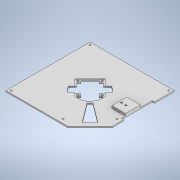
# Autodesk Inventor part: Drop_Plate
Saved by Autodesk Inventor 2022 (Build 260153000, 153)
## iProperties
Created: 2023-02-27
Part Number: Drop_Plate
Material: Generic
Document SubType Name: Modeling
Designer: zarek
Density: 1 g/cm^3
Appearance: Default
Author: zarek
Autodesk Inventor part; units mm, degrees
ref_plane "YZ Plane" through (0, 0, 0) normal (1, 0, 0) x (0, 1, 0)
ref_plane "XZ Plane" through (0, 0, 0) normal (0, 1, 0) x (-1, 0, 0)
sketch "Sketch1" plane through (0, 0, 0) normal (0, 1, 0) x (-1, 0, 0)
  line L0 (101.6, -101.6) -> (-101.6, -101.6)
  line L1 (-101.6, -101.6) -> (-101.6, 101.6)
  line L2 (-101.6, 101.6) -> (101.6, 101.6)
  line L3 (101.6, 101.6) -> (101.6, -101.6)
  line L4 (96.6, -96.6) -> (-96.6, -96.6)
  line L5 (-96.6, -96.6) -> (-96.6, 96.6)
  line L6 (-96.6, 96.6) -> (96.6, 96.6)
  line L7 (96.6, 96.6) -> (96.6, -96.6)
  line L8 (101.6, 101.6) -> (-40.4, 101.6)
  circle A0 centre (0, 0) radius 88.9
  line L9 (-40.4, 101.6) -> (-101.6, 40.4)
  line L10 (-45.4, 101.6) -> (-101.6, 45.4)
  line L11 (96.6, 96.6) -> (96.6, 101.6)
  line L12 (-45.4, 101.6) -> (-35.4, 101.6)
  line L13 (-35.4, 101.6) -> (-35.4, 96.6)
  line L14 (-35.4, 96.6) -> (-45.4, 96.6)
  line L15 (-45.4, 96.6) -> (-45.4, 101.6)
  line L16 (-101.6, 39.4) -> (-39.4, 101.6)
  line L17 (95.6, -95.6) -> (-95.6, -95.6)
  line L18 (-95.6, -95.6) -> (-95.6, 95.6)
  line L19 (-95.6, 95.6) -> (95.6, 95.6)
  line L20 (95.6, 95.6) -> (95.6, -95.6)
  point P0 (96.6, 51.2168)
  point P1 (101.6, 40.4)
  point P2 (101.6, -40.4)
  point P3 (96.6, -51.2168)
  point P4 (-96.6, 45.4)
  point P5 (-45.4, 96.6)
  point P6 (-45.4, 95.6)
  point P7 (-95.6, 45.4)
  dimension "d0" = 203.2
  dimension "d1" = 203.2
  dimension "d2" = 101.6
  dimension "d3" = 101.6
  dimension "d4" = 5
  dimension "d5" = 5
  dimension "d6" = 5
  dimension "d7" = 5
  dimension "d8" = 142
  dimension "d9" = 61.2
  dimension "d10" = 177.8
  dimension "d11" = 5
  dimension "d12" = 5
  dimension "d13" = 10
  dimension "d14" = 1
  dimension "d15" = 1
  dimension "d16" = 1
  dimension "d17" = 1
  dimension "d18" = 1
  constraints: 42 end point, 10 parallel, 8 point on line, 5 perpendicular, 4 horizontal, 1 centre point, 1 coincident
  measures "d0" distance between parallel lines of L2 L0
  measures "d1" distance between parallel lines of L1 L3
  measures "d2" distance from line of L0 point (0, 0)
  measures "d3" distance from line of L1 point (0, 0)
  measures "d4" distance between parallel lines of L4 L0
  measures "d5" distance between parallel lines of L1 L5
  measures "d6" distance between parallel lines of L2 L6
  measures "d7" distance between parallel lines of L3 L7
  measures "d8" distance of L2.end L8.end
  measures "d9" distance from line of L1 L8.end
  measures "d10" diameter of A0
  measures "d11" distance of L10.end L9.end
  measures "d12" distance of L10.start L8.end
  measures "d13" distance of L13.end L14.end
  measures "d14" distance of L9.end L16.start
  measures "d15" distance between parallel lines of L5 L18
  measures "d16" distance between parallel lines of L4 L17
  measures "d17" distance between parallel lines of L7 L20
  measures "d18" distance between parallel lines of L6 L19
extrude "Extrusion1" add sketch "Sketch1" along normal blind 3 contours L16 L19 L20 L17 L18 | A0
sketch "Sketch2" plane through (0, 3, 0) normal (0, 1, 0) x (1, 0, 0)
  circle A0 centre (0, 0) radius 34.925
  circle A1 centre (0, 0) radius 88.9
  line L0 (0, 0) -> (53.5014, -70.9987)
  line L1 (0, 0) -> (70.9987, -53.5014)
  line L2 (45.4, -95.6) -> (95.6, -45.4) projected
  line L3 (70.5, -70.5) -> (0, 0)
  point P0 (21.0184, -27.8923)
  point P1 (27.8923, -21.0184)
  dimension "d21" = 69.85
  dimension "d22" = 177.8
  dimension "d23" = 8
  dimension "d24" = 8
  constraints: 6 end point, 2 centre point, 2 coincident, 2 point on circle, 1 midpoint, 1 perpendicular
  measures "d21" diameter of A0
  measures "d22" diameter of A1
  measures "d23" angle of L1 L3
  measures "d24" angle of L0 L3
extrude "Extrusion2" cut sketch "Sketch2" against normal blind 5 contours A0 L3 A1 L0 | L1 A1 L3 A0
sketch "Sketch3" plane through (0, 3, 0) normal (0, 1, 0) x (1, 0, 0)
  circle A0 centre (0, 0) radius 2.5
  line L0 (11.3314, 2.139) -> (-2.139, -11.3314)
  line L1 (0, 0) -> (-5.6569, 5.6569)
  line L2 (-5.6569, -14.8492) -> (-26.163, 5.6569)
  line L3 (-5.6569, 26.163) -> (14.8492, 5.6569)
  circle A1 centre (-5.6569, 5.6569) radius 14
  line L4 (-26.163, 5.6569) -> (-5.6569, 26.163)
  line L5 (14.8492, 5.6569) -> (-5.6569, -14.8492)
  line L6 (-40.3051, 5.6569) -> (-5.6569, 40.3051)
  line L7 (-5.6569, 40.3051) -> (28.9914, 5.6569)
  line L8 (28.9914, 5.6569) -> (-5.6569, -28.9914)
  line L9 (-5.6569, -28.9914) -> (-40.3051, 5.6569)
  line L10 (-22.6451, 9.1747) -> (-9.1747, 22.6451)
  line L11 (-9.1747, 22.6451) -> (-12.7668, 26.2372)
  line L12 (-12.7668, 26.2372) -> (-26.2372, 12.7668)
  line L13 (-26.2372, 12.7668) -> (-22.6451, 9.1747)
  line L14 (-36.0624, 5.6569) -> (-5.6569, 36.0624)
  line L15 (-5.6569, 36.0624) -> (26.8701, 3.5355)
  line L16 (26.8701, 3.5355) -> (-3.5355, -26.8701)
  line L17 (-3.5355, -26.8701) -> (-36.0624, 5.6569)
  arc A2 (-5.6569, -28.9914) -> (28.9914, 5.6569) centre (0.4206, -0.4206) ccw
  dimension "d27" = 8
  dimension "d28" = 28
  dimension "d29" = 29
  dimension "d30" = 29
  dimension "d31" = 14.5
  dimension "d32" = 10
  dimension "d33" = 10
  dimension "d34" = 10
  dimension "d35" = 10
  dimension "d36" = 5.08
  dimension "d37" = 9.525
  dimension "d38" = 9.525
  dimension "d39" = 3
  dimension "d40" = 3
  dimension "d41" = 0
  dimension "d42" = 3
  dimension "d51" = 29.21
  constraints: 36 end point, 8 parallel, 4 perpendicular, 3 centre point, 2 coincident, 2 point on circle, 2 point on line
  measures "d27" distance of L1.start L1.end
  measures "d28" diameter of A1
  measures "d29" distance between parallel lines of L5 L4
  measures "d30" distance between parallel lines of L3 L2
  measures "d31" distance from line of A1.centre L4
  measures "d32" distance between parallel lines of L7 L3
  measures "d33" distance between parallel lines of L4 L6
  measures "d34" distance between parallel lines of L9 L2
  measures "d35" distance between parallel lines of L8 L5
  measures "d36" distance between parallel lines of L10 L12
  measures "d37" distance from line of A1.centre L11
  measures "d38" distance from line of L1.end L13
  measures "d39" distance between parallel lines of L14 L6
  measures "d40" distance between parallel lines of L9 L17
  measures "d41" distance between parallel lines of L8 L16
  measures "d42" distance between parallel lines of L7 L15
  measures "d51" radius of A2
extrude "Extrusion3" cut sketch "Sketch3" against normal blind 1 contours A0 | L0 L5 L2 L4 L3 | L4 L13 L12 L11 | A1 | L6 L7 L8 L15 L14 L17 L9 | L8 A2 | L17 L14 L15 L8
sketch "Sketch4" plane through (0, 2, 0) normal (0, 1, 0) x (1, 0, 0)
  line L0 (-36.0624, 5.6569) -> (-5.6569, 36.0624)
  line L1 (-5.6569, 36.0624) -> (26.8701, 3.5355)
  line L2 (26.8701, 3.5355) -> (-3.5355, -26.8701)
  line L3 (-3.5355, -26.8701) -> (-36.0624, 5.6569)
  line L4 (-5.6569, 40.3051) -> (28.9914, 5.6569) projected
  line L5 (-40.3051, 5.6569) -> (-5.6569, 40.3051) projected
  line L6 (-5.6569, -28.9914) -> (-40.3051, 5.6569) projected
  line L7 (28.9914, 5.6569) -> (-5.6569, -28.9914) projected
  arc A0 (-3.5355, -26.8701) -> (26.8701, 3.5355) centre (4.0877, -4.0877) ccw
  point P0 (0, 0)
  dimension "d45" = 3
  dimension "d46" = 3
  dimension "d47" = 3
  dimension "d48" = 0
  constraints: 8 end point, 2 parallel, 2 point on circle, 1 centre point, 1 perpendicular, 1 other
  measures "d45" distance between parallel lines of L4 L1
  measures "d46" distance between parallel lines of L0 L5
  measures "d47" distance between parallel lines of L6 L3
  measures "d48" distance between parallel lines of L7 L2
extrude "Extrusion4" cut sketch "Sketch4" against normal blind 5 contours L0 L1 L2 L3 | L2 A0
sketch "Sketch6" plane through (0, 3, 0) normal (0, 1, 0) x (1, 0, 0)
  line L0 (95.6, 95.6) -> (-95.6, 95.6) projected
  line L1 (95.6, 95.6) -> (90.6, 95.6)
  line L2 (90.6, 95.6) -> (90.6, -46.4)
  line L3 (90.6, -46.4) -> (95.6, -46.4)
  line L4 (95.6, -46.4) -> (95.6, 95.6)
  line L5 (95.6, -45.4) -> (95.6, 95.6) projected
  line L6 (90.6, -19.05) -> (95.6, -19.05)
  line L7 (95.6, -19.05) -> (95.6, 50.8)
  line L8 (95.6, 50.8) -> (90.6, 50.8)
  line L9 (90.6, 50.8) -> (90.6, -19.05)
  line L10 (0, 0) -> (95.6, 0)
  point P0 (95.6, -19.05)
  dimension "d58" = 5
  dimension "d59" = 142
  dimension "d62" = 50.8
  dimension "d63" = 19.05
  constraints: 18 end point, 4 parallel, 3 perpendicular, 3 point on line, 2 horizontal
  measures "d58" distance of L3.end L2.end
  measures "d59" distance between parallel lines of L3 L0
  measures "d62" distance between parallel lines of L10 L8
  measures "d63" distance between parallel lines of L10 L6
extrude "Extrusion6" cut sketch "Sketch6" against normal blind 25.4 contours L4 L10 L2 L8 | L4 L6 L2 L10
sketch "Sketch7" plane through (0, 3, 0) normal (0, 1, 0) x (1, 0, 0)
  line L0 (-95.6, 95.6) -> (-95.6, -95.6) projected
  line L1 (-95.6, -95.6) -> (45.4, -95.6) projected
  line L2 (95.6, 50.8) -> (90.6, 50.8) projected
  line L3 (90.6, 50.8) -> (65.2, 50.8)
  line L4 (90.6, -19.05) -> (90.6, 50.8)
  line L5 (90.6, -19.05) -> (90.6, 50.8) projected
  line L6 (90.6, 50.8) -> (95.6, 50.8) projected
  line L7 (90.6, 50.8) -> (59.8886, 50.8)
  line L8 (59.8886, 50.8) -> (59.8886, -10.16)
  line L9 (59.8886, -10.16) -> (90.6, -10.16)
  line L10 (90.6, -10.16) -> (90.6, 50.8)
  line L11 (59.8886, 23.8506) -> (90.6, 23.8506)
  point P0 (0, 0)
  point P1 (62.2, 50.8)
  dimension "d72" = 60.96
  dimension "d90" = 34.0106
  dimension "d154" = 30.7114
  constraints: 14 end point, 3 horizontal, 2 parallel, 2 point on line, 1 perpendicular
  measures "d72" distance of L8.end L7.end
  measures "d90" distance between parallel lines of L9 L11
  measures "d154" distance between parallel lines of L8 L4
extrude "Extrusion7" add sketch "Sketch7" along normal blind 5 contours L4 L9 L8 L11
sketch "Sketch8" plane through (0, 8, 0) normal (0, 1, 0) x (1, 0, 0)
  line L0 (59.8886, -10.16) -> (90.6, -10.16) projected
  line L1 (59.8886, -10.16) -> (90.6, -10.16)
  line L2 (90.6, -10.16) -> (90.6, 6.8326)
  line L3 (90.6, 50.8) -> (90.6, -19.05) projected
  line L4 (90.6, 6.8326) -> (65.2, 6.8326)
  circle A0 centre (74.9, 6.8326) radius 1.5
  circle A1 centre (64.8924, 6.8326) radius 1.5
  line L5 (59.8886, 23.8506) -> (59.8886, -10.16) projected
  point P0 (0, 0)
  dimension "d78" = 16.9926
  dimension "d79" = 3
  dimension "d80" = 3
  dimension "d139" = 5.0038
  dimension "d140" = 10.0076
  dimension "d153" = 15.7
  constraints: 6 end point, 3 point on line, 2 centre point, 1 collinear, 1 perpendicular, 1 other
  measures "d78" distance of L0.end L2.end
  measures "d79" diameter of A0
  measures "d80" diameter of A1
  measures "d140" distance of A0.centre A1.centre
  measures "d153" distance from line of L3 A0.centre
hole "Hole1" at (74.9, 8, -6.8326) at (64.8924, 8, -6.8326) direction (0, -1, 0) diameter 2.85 depth 5.08 tip angle 118 countersink diameter 3.81 countersink angle 82 thread size "M3.5x0.6" class "6H" standard "ANSI Metric M Profile"
sketch "Sketch9" plane through (0, 2, 0) normal (0, 1, 0) x (1, 0, 0)
  point P0 (0, 0)
sketch "Sketch10" plane through (0, 2, 0) normal (0, 1, 0) x (1, 0, 0)
  circle A0 centre (6.7129, 18.0166) radius 2
  circle A1 centre (-18.0312, -6.7275) radius 2
  circle A2 centre (-18.0312, -6.7275) radius 2
  circle A3 centre (-5.6569, 5.6469) radius 14
  circle A4 centre (0, -0.01) radius 2.5
  circle A5 centre (22.2964, 5.2615) radius 2.2448
  circle A6 centre (-5.2761, -22.3111) radius 2.3104
  circle A7 centre (-33.9469, 6.3598) radius 2.2008
  circle A8 centre (-6.3744, 33.9323) radius 2.3894
  line L0 (-5.6569, 40.3051) -> (28.9914, 5.6569) projected
  line L1 (-5.6569, 40.3051) -> (1.4142, 33.234)
  line L2 (-5.6569, 26.163) -> (1.4142, 33.234)
  line L3 (-5.6569, 26.163) -> (-12.7279, 33.234)
  line L4 (-40.3051, 5.6569) -> (-5.6569, 40.3051) projected
  line L5 (-5.6569, 40.3051) -> (-40.3051, 5.6569)
  line L6 (-5.6569, 26.163) -> (-33.234, -1.4142)
  line L7 (-5.6569, -28.9914) -> (-40.3051, 5.6569) projected
  line L8 (-33.234, 12.7279) -> (-26.163, 5.6569)
  arc A9 (-5.6569, -28.9914) -> (21.0752, -21.0752) centre (0.4206, -0.4206) ccw projected
  line L9 (-5.6569, -28.9914) -> (28.9914, 5.6569)
  line L10 (-5.6569, 36.0624) -> (26.8701, 3.5355) projected
  line L11 (-12.7279, -21.9203) -> (21.9203, 12.7279)
  line L12 (-5.6569, -14.8492) -> (1.4142, -21.9203)
  line L13 (14.8492, 5.6569) -> (21.9203, -1.4142)
  point P0 (0, 0)
  point P1 (0.0071, -0.017)
  point P2 (24.4219, 5.9837)
  point P3 (23.0187, 7.3869)
  point P4 (19.799, 10.6066)
  dimension "d91" = 34.9934
  dimension "d92" = 28
  dimension "d93" = 8
  dimension "d94" = 10
  dimension "d95" = 10
  dimension "d96" = 10
  dimension "d97" = 10
  dimension "d98" = 10
  constraints: 20 end point, 11 point on line, 9 centre point, 7 perpendicular, 2 coincident, 1 collinear
  measures "d91" distance of A2.centre A0.centre
  measures "d92" diameter of A3
  measures "d93" distance of point (-5.657, 5.647) A4.centre
  measures "d94" distance between parallel lines of L3 L0
  measures "d95" distance between parallel lines of L2 L4
  measures "d96" distance between parallel lines of L7 L8
  measures "d97" distance between parallel lines of L4 L6
  measures "d98" distance between parallel lines of L13 L0
extrude "Extrusion8" add sketch "Sketch10" against normal up to surface (2 mm away) contours A5 L10 L9 L13 L11 | L2 L3 L4 L0 | L9 L7 L11 L12 | L6 L7 L4 L8
sketch "Sketch11" plane through (0, 3, 0) normal (0, 1, 0) x (1, 0, 0)
  circle A0 centre (6.7129, 18.0166) radius 2
  circle A1 centre (-18.0312, -6.7275) radius 2
  circle A2 centre (-18.0312, -6.7275) radius 2
  circle A3 centre (-5.6569, 5.6469) radius 14
  circle A4 centre (0, -0.01) radius 2.5
  circle A5 centre (22.2964, 5.2615) radius 2.2448
  circle A6 centre (-5.2761, -22.3111) radius 2.3104
  circle A7 centre (-33.9469, 6.3598) radius 2.2008
  circle A8 centre (-6.3744, 33.9323) radius 2.3894
  line L0 (-5.6569, 40.3051) -> (28.9914, 5.6569)
  line L1 (-5.6569, 40.3051) -> (1.4142, 33.234)
  line L2 (-5.6569, 26.163) -> (1.4142, 33.234)
  line L3 (-5.6569, 26.163) -> (-12.7279, 33.234)
  line L4 (-40.3051, 5.6569) -> (-5.6569, 40.3051)
  line L5 (-5.6569, 40.3051) -> (-40.3051, 5.6569)
  line L6 (-5.6569, 26.163) -> (-33.234, -1.4142)
  line L7 (-5.6569, -28.9914) -> (-40.3051, 5.6569)
  line L8 (-33.234, 12.7279) -> (-26.163, 5.6569)
  arc A9 (-5.6569, -28.9914) -> (21.0752, -21.0752) centre (0.4206, -0.4206) ccw
  line L9 (-5.6569, -28.9914) -> (28.9914, 5.6569)
  line L10 (-5.6569, 36.0624) -> (26.8701, 3.5355)
  line L11 (-12.7279, -21.9203) -> (21.9203, 12.7279)
  line L12 (-5.6569, -14.8492) -> (1.4142, -21.9203)
  line L13 (14.8492, 5.6569) -> (21.9203, -1.4142)
  point P0 (0, 0)
  point P1 (0, 0)
  point P2 (0.0071, -0.017)
  point P3 (24.4219, 5.9837)
  point P4 (23.0187, 7.3869)
  point P5 (19.799, 10.6066)
  point P6 (24.4219, 5.9837)
  point P7 (23.0187, 7.3869)
  dimension "d101" = 34.9934
  dimension "d102" = 28
  dimension "d103" = 8
  dimension "d104" = 10
  dimension "d105" = 10
  dimension "d106" = 10
  dimension "d107" = 10
  dimension "d108" = 10
  constraints: 28 end point, 11 point on line, 10 centre point, 7 perpendicular, 2 coincident, 2 point on circle, 1 collinear
  measures "d101" distance of A2.centre A0.centre
  measures "d102" diameter of A3
  measures "d103" distance of point (-5.657, 5.647) A4.centre
  measures "d104" distance between parallel lines of L3 L0
  measures "d105" distance between parallel lines of L2 L4
  measures "d106" distance between parallel lines of L7 L8
  measures "d107" distance between parallel lines of L4 L6
  measures "d108" distance between parallel lines of L13 L0
extrude "Extrusion9" cut sketch "Sketch11" against normal blind 10 contours A5 L10 | A6 | A7 | A8 picked at (21.4653, 4.9881)
sketch "Sketch12" plane through (0, 3, 0) normal (0, 1, 0) x (1, 0, 0)
  line L0 (95.6, 50.8) -> (95.6, 95.6) projected
  line L1 (-95.6, -95.6) -> (45.4, -95.6) projected
  line L2 (95.6, 95.6) -> (-95.6, -95.6)
  line L3 (95.6, 95.6) -> (-95.6, 95.6) projected
  line L4 (0, 95.6) -> (0, -95.6)
  line L5 (-95.6, -95.6) -> (45.4, -95.6) projected
  point P0 (0, 0)
  constraints: 4 end point, 1 midpoint, 1 point on line, 1 vertical
ref_plane "Work Plane2" through (0, 3, -95.6) normal (-1, 0, 0) x (0, 0, 1)
sketch "Sketch15" plane through (0, 3, 0) normal (0, 1, 0) x (1, 0, 0)
  line L0 (-96.6, 96.6) -> (-96.6, -96.6)
  line L1 (96.6, 96.6) -> (-96.6, 96.6)
  line L2 (-96.6, 96.6) -> (96.6, 96.6)
  line L3 (96.6, -45.4) -> (45.4, -96.6)
  line L4 (96.6, 96.6) -> (96.6, -45.4)
  line L5 (96.6, -45.4) -> (45.4, -96.6)
  line L6 (45.4, -96.6) -> (-96.6, -96.6)
  line L7 (-96.6, -96.6) -> (-96.6, 96.6)
  line L8 (-96.6, 96.6) -> (-89.5289, 89.5289)
  circle A0 centre (-89.5289, 89.5289) radius 5
  circle A1 centre (-89.5289, 89.5289) radius 1.5
  line L9 (-89.5289, 84.5289) -> (-96.6, 84.5289)
  line L10 (-89.5289, 89.5289) -> (-89.5289, 84.5289)
  line L11 (-89.5289, 89.5289) -> (-84.5289, 89.5289)
  line L12 (-84.5289, 96.6) -> (-84.5289, 89.5289)
  line L13 (-96.6, -96.6) -> (-89.5289, -89.5289)
  line L14 (-96.6, -96.6) -> (-86.6, -96.6) construction
  circle A2 centre (-89.5289, -89.5289) radius 5
  circle A3 centre (-89.5289, -89.5289) radius 1.75
  line L15 (-89.5289, -89.5289) -> (-84.5289, -89.5289)
  line L16 (-84.5289, -96.6) -> (-84.5289, -89.5289)
  line L17 (-89.5289, -89.5289) -> (-89.5289, -84.5289)
  line L18 (-96.6, -84.5289) -> (-89.5289, -84.5289)
  line L19 (96.6, 96.6) -> (89.5289, 89.5289)
  circle A4 centre (89.5289, 89.5289) radius 5
  circle A5 centre (89.5289, 89.5289) radius 1.75
  line L20 (89.5289, 89.5289) -> (84.5289, 89.5289)
  line L21 (84.5289, 96.6) -> (84.5289, 89.5289)
  line L22 (89.5289, 89.5289) -> (89.5289, 84.5289)
  line L23 (96.6, 84.5289) -> (89.5289, 84.5289)
  line L24 (96.6, -43.114) -> (96.6, 96.6)
  line L25 (-96.6, -96.6) -> (43.1178, -96.6)
  line L26 (28.9914, 5.6569) -> (-5.6569, -28.9914)
  line L27 (25.4, -25.4) -> (101.6, -25.4)
  line L28 (101.6, -88.9) -> (101.6, 101.6)
  line L29 (25.4, -25.4) -> (25.4, -101.6)
  line L30 (43.1178, -101.6) -> (-101.6, -101.6)
  line L31 (96.6, -25.4) -> (86.6, -25.4)
  circle A6 centre (86.6, -25.4) radius 5
  circle A7 centre (86.6, -25.4) radius 1.75
  line L32 (25.4, -96.6) -> (25.4, -86.6)
  circle A8 centre (25.4, -86.6) radius 5
  circle A9 centre (25.4, -86.6) radius 1.75
  point P0 (0, 0)
  point P1 (0, 0)
  dimension "d117" = 10
  dimension "d118" = 3
  dimension "d119" = 10
  dimension "d120" = 45
  dimension "d121" = 10
  dimension "d122" = 3.5
  dimension "d123" = 10
  dimension "d124" = 10
  dimension "d125" = 3.5
  dimension "d126" = 76.2
  dimension "d127" = 76.2
  dimension "d128" = 10
  dimension "d129" = 10
  dimension "d130" = 3.5
  dimension "d131" = 10
  dimension "d132" = 10
  dimension "d133" = 3.5
  constraints: 66 end point, 14 point on line, 10 centre point, 9 coincident, 9 perpendicular, 6 point on circle, 5 horizontal, 3 parallel, 2 tangent, 1 collinear, 1 equal length, 1 vertical
  measures "d117" distance of L0.start L8.end
  measures "d118" diameter of A1
  measures "d119" distance of L6.end L13.end
  measures "d120" angle of L14 L13
  measures "d121" diameter of A2
  measures "d122" diameter of A3
  measures "d123" distance of L1.start L19.end
  measures "d124" diameter of A4
  measures "d125" diameter of A5
  measures "d126" distance between parallel lines of L28 L29
  measures "d127" distance between parallel lines of L30 L27
  measures "d128" distance of L31.start L31.end
  measures "d129" diameter of A6
  measures "d130" diameter of A7
  measures "d131" distance of L32.start L32.end
  measures "d132" diameter of A8
  measures "d133" diameter of A9
extrude "Extrusion12" cut sketch "Sketch15" against normal blind 25.4 contours A1 L11 L8 | L8 L10 A1 | L10 L11 A1 | L17 L13 A3 | A3 L15 L17 | L20 L22 A5 | A5 L19 L20 | L13 L15 A3 | A5 L22 L19 | A9 L29 | L29 A9 | A7 L27 | L27 A7
sketch "Sketch18" plane through (0, 3, 0) normal (0, 1, 0) x (1, 0, 0)
  circle A0 centre (0, 0) radius 38.1
  circle A1 centre (0, 0) radius 36.35
  line L0 (-0.7071, 31.1127) -> (19.799, 10.6066) projected
  line L1 (6.364, 24.0416) -> (11.387, 29.0647)
  line L2 (24.8221, 15.6297) -> (19.799, 10.6066)
  line L3 (6.364, 24.0416) -> (19.799, 10.6066)
  line L4 (19.799, 10.6066) -> (14.8492, 5.6569) projected
  line L5 (-5.6569, 26.163) -> (-0.7071, 31.1127) projected
  line L6 (11.387, 29.0647) -> (15.297, 32.9746)
  line L7 (24.8221, 15.6297) -> (29.8595, 20.7299)
  line L8 (15.297, 32.9746) -> (-32.9746, -15.297)
  line L9 (29.8595, 20.7299) -> (-20.7299, -29.8595)
  line L10 (-5.6569, -14.8492) -> (-10.6066, -19.799) projected
  line L11 (-10.6066, -19.799) -> (-24.0416, -6.364)
  point P0 (-20.7299, -29.8595)
  point P1 (-10.638, -19.7676)
  dimension "d147" = 76.2
  dimension "d148" = 72.7
  dimension "d149" = 0
  dimension "d150" = 10
  constraints: 14 end point, 5 point on line, 4 point on circle, 2 centre point, 2 coincident, 2 perpendicular, 1 collinear, 4 other
  measures "d147" diameter of A0
  measures "d148" diameter of A1
  measures "d149" distance between parallel lines of L4 L2
  measures "d150" distance between parallel lines of L1 L5
extrude "Extrusion15" cut sketch "Sketch18" against normal blind 25.4 contours L9 L0 L1 L6 A1 | L7 L2 L0 L9 | A1 L8 L11 L9
equation "\"d1\" = d0"
equation "\"d2\" = 0.5 * d0"
equation "\"d3\" = 0.5 * d0"
body "Solid1"
